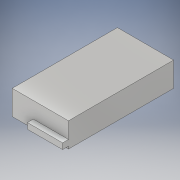
# Autodesk Inventor part: S-201-24
Saved by Autodesk Inventor 2019.4 (Build 234330000, 330)
## iProperties
Created: 2021-02-08
Part Number: S-201-24
Material: Generic
Document SubType Name: Modeling
Designer: Jorian Brusind
Density: 1 g/cm^3
Appearance: Aluminum - Polished
Author: Jorian Brusind
Autodesk Inventor part; units mm, degrees
ref_plane "YZ Plane" through (0, 0, 0) normal (1, 0, 0) x (0, 1, 0)
ref_plane "XZ Plane" through (0, 0, 0) normal (0, 1, 0) x (-1, 0, 0)
ref_plane "XY Plane" through (0, 0, 0) normal (0, 0, 1) x (1, 0, 0)
sketch "Sketch1" plane through (0, 0, 0) normal (0, 1, 0) x (-1, 0, 0)
  line L0 (0, 0) -> (115, 0)
  line L1 (115, 0) -> (115, -215)
  line L2 (115, -215) -> (0, -215)
  line L3 (0, -215) -> (0, 0)
  dimension "d0" = 115
  dimension "d1" = 215
  constraints: 8 end point, 2 parallel, 1 horizontal, 1 perpendicular
  measures "d0" distance of L1.end L2.end
  measures "d1" distance of L0.end L1.end
extrude "Extrusion1" add sketch "Sketch1" along normal blind 50
sketch "Sketch2" plane through (-115, 0, 0) normal (0, 0, 1) x (1, 0, 0)
  line L0 (115, 0) -> (115, 5)
  line L1 (115, 0) -> (115, 50) projected
  line L2 (115, 5) -> (43, 5)
  line L3 (43, 5) -> (43, 17)
  line L4 (43, 17) -> (115, 17)
  line L5 (115, 17) -> (115, 5)
  dimension "d4" = 5
  dimension "d5" = 72
  dimension "d6" = 12
  constraints: 10 end point, 2 parallel, 1 horizontal, 1 perpendicular, 1 point on line
  measures "d4" distance of L0.start L0.end
  measures "d5" distance of L3.end L4.end
  measures "d6" distance of L2.end L3.end
extrude "Extrusion2" add sketch "Sketch2" along normal blind 12
body "Solid1"
